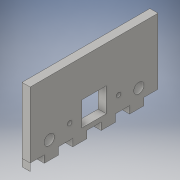
# Autodesk Inventor part: Part15
Saved by Autodesk Inventor 2016 (Build 200138000, 138)
## iProperties
Created: 2018-01-18
Part Number: Part15
Material: Generic
Document SubType Name: Modeling
Designer: student
Density: 1 g/cm^3
Appearance: Default
Author: student
Autodesk Inventor part; units mm, degrees
ref_plane "YZ Plane" through (0, 0, 0) normal (1, 0, 0) x (0, 1, 0)
ref_plane "XZ Plane" through (0, 0, 0) normal (0, 1, 0) x (-1, 0, 0)
ref_plane "XY Plane" through (0, 0, 0) normal (0, 0, 1) x (1, 0, 0)
ref_plane "Work Plane1" through (-108.8053, -23.2276, 20.9918) normal (0, 1, 0) x (-0.9999918, 0, -0.00406)
sketch "Sketch1" plane through (-108.8053, -23.2276, 20.9918) normal (0, 1, 0) x (-0.9999918, 0, -0.00406)
  line L0 (-46.787, -50.1863) -> (-47.193, 49.8137)
  line L1 (-47.193, 49.8137) -> (-40.843, 49.8137)
  line L2 (-46.787, -50.1863) -> (-40.437, -50.1863)
  line L3 (-46.787, -50.1863) -> (-40.437, -50.1863)
  line L4 (-40.843, 49.8137) -> (-40.437, -50.1863)
  line L5 (-47.193, 49.8137) -> (46.787, 50.1953) construction
  line L6 (-38.1849, 20.7247) -> (-38.1707, 17.2247)
  line L7 (-38.0296, -17.525) -> (-38.0154, -21.025)
  point P0 (-108.7192, -21.4334)
  dimension "d0" = 6.35
  dimension "d1" = 6.35
  constraints: 14 end point, 3 horizontal, 1 coincident, 1 collinear, 6 other
  measures "d0" distance of L0.end L1.end
  measures "d1" distance of L0.start L2.end
extrude "Extrusion1" add sketch "Sketch1" along normal blind 50.8 and the other way blind 6.35
sketch "Sketch2" plane through (-61.8149, -29.5776, 70.9967) normal (1, 0, 0) x (0, 0, -1)
  line L0 (100.0008, 0) -> (100.0008, 57.15) construction
  line L1 (0, 57.15) -> (100.0008, 57.15) construction
  line L2 (0, 0) -> (0, 57.15) construction
  line L3 (0, 57.15) -> (100.0008, 57.15) construction
  line L4 (50.0004, 57.15) -> (50.0004, 0) construction
  circle A0 centre (15.0004, 13.9978) radius 4
  circle A1 centre (85.0004, 13.9978) radius 4
  line L5 (40.4004, 9.271) -> (59.6004, 9.271)
  line L6 (59.6004, 9.271) -> (59.6004, 28.291)
  line L7 (59.6004, 28.291) -> (40.4004, 28.291)
  line L8 (40.4004, 28.291) -> (40.4004, 9.271)
  line L9 (21.3504, 9.271) -> (21.3504, 25.4) construction
  line L10 (21.3504, 20.3478) -> (13.3504, 20.3478) construction
  line L11 (21.3504, 9.271) -> (21.3504, 25.4) projected
  line L12 (78.6504, 9.271) -> (78.6504, 25.4) projected
  line L13 (11.1112, 0) -> (11.1112, 5.715)
  line L14 (22.2224, 5.715) -> (22.2224, 0)
  line L15 (33.3334, 0) -> (33.3334, 5.715)
  line L16 (44.4446, 5.715) -> (44.4446, 0)
  line L17 (55.5556, 0) -> (55.5556, 5.715)
  line L18 (66.6668, 5.715) -> (66.6668, 0)
  line L19 (88.8891, 5.715) -> (88.8891, 0)
  line L20 (77.7779, 0) -> (77.7779, 5.715)
  line L21 (88.8891, 5.715) -> (100.0008, 5.715) construction
  line L22 (0.0258, 0) -> (0.0258, 5.715) construction
  line L23 (0.0258, 57.15) -> (0.0258, 0) construction
  line L24 (88.8891, 0) -> (100.0266, 0)
  line L25 (100.0008, 5.715) -> (88.8891, 5.715)
  line L26 (77.7779, 0) -> (66.6668, 0)
  line L27 (66.6668, 5.715) -> (77.7779, 5.715)
  line L28 (55.5556, 0) -> (44.4446, 0)
  line L29 (44.4446, 5.715) -> (55.5556, 5.715)
  line L30 (33.3334, 0) -> (22.2224, 0)
  line L31 (22.2224, 5.715) -> (33.3334, 5.715)
  line L32 (11.1112, 0) -> (0.0258, 0)
  line L33 (11.1112, 5.715) -> (0.0258, 5.715)
  line L34 (0.0258, 0) -> (0.0258, 5.715)
  line L35 (100.0266, 0) -> (100.0008, 5.715)
  line L36 (59.6004, 9.271) -> (59.6004, 25.4) projected
  line L37 (40.4004, 9.271) -> (40.4004, 25.4) projected
  circle A2 centre (30.8754, 17.3) radius 1.75
  circle A3 centre (69.1254, 17.3) radius 1.75
  point P0 (70.9967, 23.2276)
  point P1 (75.0381, 0)
  dimension "d9" = 8
  dimension "d10" = 8
  dimension "d13" = 35
  dimension "d14" = 8
  dimension "d26" = 5.715
  dimension "d27" = 5.715
  dimension "d28" = 5.715
  dimension "d29" = 5.715
  dimension "d30" = 5.715
  constraints: 58 end point, 7 horizontal, 4 centre point, 4 point on line, 2 parallel, 1 coincident, 1 midpoint, 1 perpendicular, 1 symmetric about line, 4 other
  measures "d9" diameter of A0
  measures "d10" diameter of A1
  measures "d13" distance from line of L4 A0.centre
  measures "d14" distance of L10.start L10.end
  measures "d26" distance of L13.start L13.end
  measures "d27" distance of L15.start L15.end
  measures "d28" distance of L17.start L17.end
  measures "d29" distance of L20.start L20.end
  measures "d30" vertical distance of L24.end L21.end
extrude "Extrusion2" cut sketch "Sketch2" against normal blind 35
equation "\"d27\" = d26"
equation "\"d28\" = d26"
equation "\"d29\" = d26"
equation "\"d30\" = d26"
equation "\"d11\" = d13"
body "Solid1"
